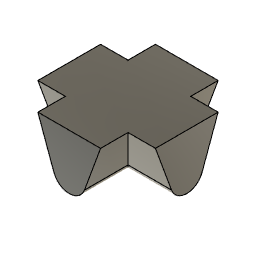
Texture example 01 model (Autodesk Fusion 360 design; units mm, degrees)
Autodesk Fusion 360 part; units mm, degrees
sketch "Skizze1" plane through (0, 0, 0) normal (0, 1, 0) x (1, 0, 0)
  line L0 (0.4, 0) -> (-0.4, 0)
  line L1 (-0.4, 0) -> (-0.1949, 0.5635)
  arc A0 (0.1949, 0.5635) -> (-0.1949, 0.5635) centre (0, 0.4926) ccw
  line L2 (0.1949, 0.5635) -> (0.4, 0)
  line L3 (0, -1.75) -> (0, -22.5)
  line L4 (1.75, 0) -> (22.5, 0) construction
  line L5 (0, 0) -> (0, 0.7) construction
  dimension "d1" = 40
  dimension "d2" = 0.8
  dimension "d3" = 0.7
  constraint tangent L1 A0
  constraint tangent A0 L2
  constraint symmetric L1 L2 L3
  constraint coincident L0.end L4
  constraint coincident L0.start L4
  constraint coincident L4 L5.start
  constraint coincident A0 L5.end
  constraint collinear L3 L5
  measures "d1" angle of L1 L2
  measures "d2" horizontal distance of L0.start L0.end
  measures "d3" vertical distance of L5.start L5.end
extrude "Extrusion1" add sketch "Skizze1" along normal mid plane 1.5 makes body 1
pattern_circular "C-Anordnung1" count 2 over 90 about axis through (0, 0, 1.75) along (0, 0, 1) of "Extrusion1" makes body 2
combine "Kombinieren1" operation add target body 1 tool bodies 2
